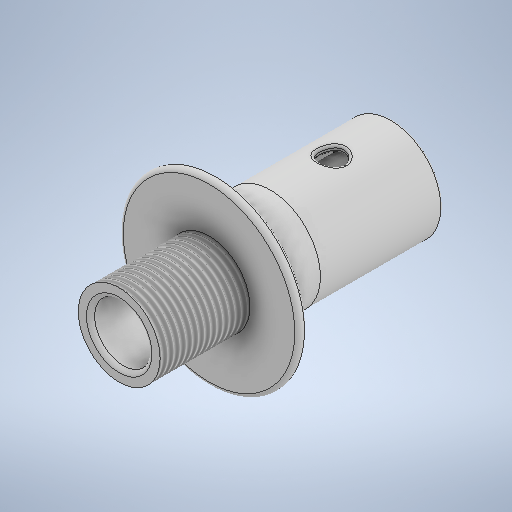
# Autodesk Inventor part: Adapter
Saved by Autodesk Inventor 2025.2 (Build 292293000, 293)
## iProperties
Created: 2025-03-09
Part Number: Adapter
Material: Generic
Document SubType Name: Modeling
Designer: eason
Density: 1 g/cm^3
Appearance: Default
Author: eason
Autodesk Inventor part; units mm, degrees
ref_plane "YZ Plane" through (0, 0, 0) normal (1, 0, 0) x (0, 1, 0)
ref_plane "XZ Plane" through (0, 0, 0) normal (0, 1, 0) x (-1, 0, 0)
ref_plane "XY Plane" through (0, 0, 0) normal (0, 0, 1) x (1, 0, 0)
sketch "Sketch1" plane through (0, 0, 0) normal (0, 0, 1) x (1, 0, 0)
  circle A0 centre (0, 0) radius 10
  circle A1 centre (0, 0) radius 12.25
  circle A2 centre (0, 0) radius 7
  dimension "d0" = 20
  dimension "d1" = 24.5
  dimension "d3" = 3
  constraints: 3 centre point, 3 coincident
  measures "d0" diameter of A0
  measures "d1" diameter of A1
  measures "d3" radial gap between concentric circles of A2 A0
extrude "Extrusion1" add sketch "Sketch1" along normal blind 22 contours A0
extrude "Extrusion2" add sketch "Sketch1" against normal blind 5 contours A0 | A1
sketch "Sketch2" plane through (0, 0, -5) normal (0, 0, -1) x (-1, 0, 0)
  circle A0 centre (0, 0) radius 12.25 projected
  circle A1 centre (0, 0) radius 10.75
  dimension "d8" = 21.5
  constraints: 1 centre point, 1 coincident
  measures "d8" diameter of A1
extrude "Extrusion3" add sketch "Sketch2" along normal blind 40
thread "Thread1" size "M20x1.5" class "6g" standard "ANSI Metric M Profile" full length
sketch "Sketch6" plane through (0, 0, 0) normal (0, 1, 0) x (-1, 0, 0)
  line L0 (12.25, 0) -> (-12.25, 0) projected
  line L1 (12.25, 0) -> (22.25, 0)
  arc A0 (20.4038, -2.7692) -> (22.25, 0) centre (19.25, 0) ccw
  line L2 (12.25, 0) -> (12.25, -45) projected
  arc A1 (20.4038, -2.7692) -> (12.25, -15) centre (25.5, -15) ccw
  line L3 (0, -54) -> (0, 9) projected
  point P0 (0, 0)
  dimension "d17" = 10
  dimension "d18" = 15
  dimension "d19" = 7
  constraints: 4 point on circle, 2 centre point, 2 end point, 2 tangent, 1 horizontal, 1 line through centre, 1 point on line
  measures "d17" distance of L0.start L1.end
  measures "d18" distance of A1.end L0.start
  measures "d19" distance of L0.start A0.centre
revolve "Revolution1" add sketch "Sketch6" angle 360 about axis through (0, 0, -10) along (0, 0, 1)
fillet "Fillet1" radius 1 1 edges at (-7, 0, 22)
fillet "Fillet2" radius 1 1 edges at (22.25, 0, 0)
sketch "Sketch7" plane through (0, 0, 0) normal (0, 1, 0) x (-1, 0, 0)
  circle A0 centre (0, -30) radius 3
  line L0 (0, -54) -> (0, 9) projected
  line L1 (-12.25, -45) -> (12.25, -45) projected
  point P0 (0, 0)
  dimension "d23" = 6
  dimension "d24" = 15
  constraints: 1 centre point, 1 point on line
  measures "d23" diameter of A0
  measures "d24" distance from line of L1 A0.centre
extrude "Extrusion4" cut sketch "Sketch7" along normal through all both and the other way through all
fillet "Fillet4" radius 0.5 4 edges at (2.9308, -10.3428, -29.3595) (2.9343, -11.8934, -29.3757) (2.9308, 10.3428, -29.3595) (2.9343, 11.8934, -29.3757)
sketch "Sketch8" plane through (0, 0, -5) normal (0, 0, -1) x (-1, 0, 0)
  circle A0 centre (0, 0) radius 8.85
  circle A1 centre (0, 0) radius 7 projected
  dimension "d29" = 17.7
  constraints: 1 centre point, 1 coincident
  measures "d29" diameter of A0
extrude "Extrusion5" add sketch "Sketch8" along normal up to surface (40 mm away)
fillet "Fillet5" radius 0.5 4 edges at (10.75, 0, -45) (12.25, 0, -45) (8.85, 0, -45) (7, 0, -45)
body "Solid1"
